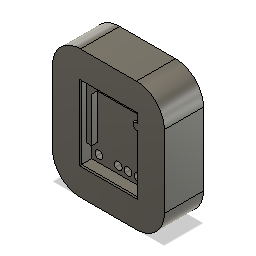
Fomu Hacker Programming Jig (Autodesk Fusion 360 design; units mm, degrees)
Autodesk Fusion 360 part; units mm, degrees
sketch "Sketch1" plane through (0, 0, 0) normal (0, 0, 1) x (1, 0, 0)
  line L0 (0, 0) -> (10, 0)
  line L1 (10, 0) -> (10, 13)
  line L2 (10, 13) -> (0, 13)
  line L3 (0, 13) -> (0, 0)
  line L4 (15, -5) -> (15, 18)
  line L5 (15, 18) -> (-5, 18)
  line L6 (-5, 18) -> (-5, -5)
  line L7 (-5, -5) -> (15, -5)
  dimension "d1" = 10
  dimension "d2" = 13
  dimension "d3" = 5
  measures "d1" distance of L0.start
  measures "d2" distance of L0.start
  measures "d3" distance of L1
extrude "Extrude1" add sketch "Sketch1" along normal blind 7
sketch "Sketch2" plane through (0, 0, 0) normal (0, 0, -1) x (-1, 0, 0)
  line L0 (0, 13) -> (0, 0)
  line L1 (0, 0) -> (-10, 0)
  line L2 (-10, 0) -> (-10, 13)
  line L3 (-10, 13) -> (0, 13)
  line L4 (-15, -5) -> (5, -5)
  line L5 (5, -5) -> (5, 18)
  line L6 (5, 18) -> (-15, 18)
  line L7 (-15, 18) -> (-15, -5)
extrude "Extrude2" add sketch "Sketch2" against normal blind 5 contours L0 L1 L2 L3
sketch "Sketch3" plane through (0, 0, 5) normal (0, 0, 1) x (1, 0, 0)
  line L0 (10, 0) -> (10, 13)
  line L1 (10, 13) -> (0, 13)
  line L2 (0, 13) -> (0, 0)
  line L3 (0, 0) -> (10, 0)
  line L4 (0, 10) -> (3, 13)
  line L5 (0, 13) -> (3, 13)
  line L6 (0, 13) -> (0, 10)
  dimension "d73" = 3
  dimension "d74" = 3
extrude "Extrude3" add sketch "Sketch3" along normal blind 1 contours L1 L2 L4 L5 L6
sketch "Sketch4" plane through (0, 0, 5) normal (0, 0, 1) x (1, 0, 0)
  line L0 (10, 13) -> (3, 13)
  line L1 (0, 10) -> (0, 0)
  line L2 (0, 0) -> (10, 0)
  line L3 (10, 0) -> (10, 13)
  circle A0 centre (1.3, 1.25) radius 0.7
  circle A1 centre (9, 8.2) radius 0.7
  circle A2 centre (9, 5.3) radius 0.7
  circle A3 centre (9, 3.3) radius 0.7
  circle A4 centre (8.35, 1.25) radius 0.7
  circle A5 centre (6.5, 1.25) radius 0.7
  circle A6 centre (4.75, 1.25) radius 0.7
  line L4 (3, 13) -> (0, 10)
  dimension "d12" = 3.3
  dimension "d14" = 5.3
  dimension "d15" = 8.2
  dimension "d16" = 1.4
  dimension "d17" = 1.4
  dimension "d18" = 1.4
  dimension "d19" = 1.25
  dimension "d21" = 1.4
  dimension "d22" = 1.4
  dimension "d23" = 1.4
  dimension "d24" = 1.4
  dimension "d68" = 1
  dimension "d69" = 1.65
  dimension "d70" = 3.5
  dimension "d71" = 5.25
  dimension "d72" = 8.7
  measures "d12" distance of L1.end
  measures "d14" distance of L1.end
  measures "d15" distance of L1.end
  measures "d16" diameter of A3
  measures "d17" diameter of A2
  measures "d18" diameter of A1
  measures "d19" distance of L1.end
  measures "d21" diameter of A4
  measures "d22" diameter of A5
  measures "d23" diameter of A6
  measures "d24" diameter of A0
extrude "Extrude4" cut sketch "Sketch4" against normal blind 8.5 contours A0 | A1 | A2 | A3 | A4 | A5 | A6
sketch "Sketch6" plane through (0, 0, 7) normal (0, 0, 1) x (1, 0, 0)
  line L0 (-5, -5) -> (15, -5)
  line L1 (15, -5) -> (15, 18)
  line L2 (15, 18) -> (-5, 18)
  line L3 (-5, 18) -> (-5, -5)
  line L4 (0, 0) -> (0, 13)
  line L5 (0, 13) -> (10, 13)
  line L6 (10, 13) -> (10, 0)
  line L7 (10, 0) -> (0, 0)
  arc A0 (10, 11.75) -> (10, 10.25) centre (10, 11) ccw
  line L8 (10, 11.75) -> (10, 10.25)
  dimension "d63" = 1.5
  dimension "d64" = 11
  measures "d63" diameter of A0
extrude "Extrude6" add sketch "Sketch6" against normal blind 2 contours L6 A0 L8
chamfer "Chamfer2" distance 0.2 angle 45 6 edges at (5, 13, 7) (10, 12.375, 7) (9.25, 11, 7) (10, 5.125, 7) (5, 0, 7) (0, 6.5, 7)
fillet "Fillet3" radius 5 4 edges at (-5, -5, 3.5) (15, -5, 3.5) (-5, 18, 3.5) (15, 18, 3.5)
sketch "Sketch7" plane through (0, 0, 5) normal (0, 0, 1) x (1, 0, 0)
  arc A0 (10, 11.75) -> (10, 10.25) centre (10, 11) ccw
  line L0 (10, 11.75) -> (10, 13)
  line L1 (10, 13) -> (3, 13)
  line L2 (3, 13) -> (0, 10)
  line L3 (0, 10) -> (0, 0)
  line L4 (0, 0) -> (10, 0)
  line L5 (10, 0) -> (10, 10.25)
  circle A1 centre (6.5, 1.25) radius 0.7
  circle A2 centre (9, 8.2) radius 0.7
  circle A3 centre (8.35, 1.25) radius 0.7
  circle A4 centre (4.75, 1.25) radius 0.7
  circle A5 centre (9, 5.3) radius 0.7
  circle A6 centre (9, 3.3) radius 0.7
  circle A7 centre (1.3, 1.25) radius 0.7
  line L6 (2, 12) -> (10, 12)
  line L7 (1, 11) -> (1, 3)
  line L8 (1, 3) -> (0, 3)
  line L9 (0, 13) -> (10, 13)
  dimension "d76" = 1
  dimension "d77" = 1
  dimension "d78" = 10
  measures "d76" distance of L1 L6
  measures "d77" distance of L3 L7
  measures "d78" distance of L8 L9
extrude "Extrude7" add sketch "Sketch7" along normal blind 1 contours L0 L1 L2 L6 L9 | L2 L3 L7 L8
chamfer "Chamfer3" distance 1 angle 45 7 edges at (0.6474, 0.9969, 0) (4.0974, 0.9969, 0) (5.8474, 0.9969, 0) (7.6974, 0.9969, 0) (8.3474, 3.0469, 0) (8.3474, 5.0469, 0) (8.3474, 7.9469, 0)
equation "d16 = d18"
equation "d17 = d18"
equation "d21 = d18"
equation "d22 = d18"
equation "d23 = d18"
equation "d24 = d18"
